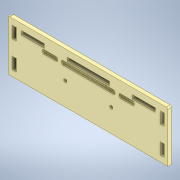
# Autodesk Inventor part: case bottom front
Saved by Autodesk Inventor 2022.3 (Build 263350030, 350C)
## iProperties
Created: 2021-05-28
Part Number: case bottom front
Material: Nylon, molybdenum disulphide
Document SubType Name: Modeling
Designer: benka
Density: 1.13 g/cm^3
Appearance: Nylon 6
Author: benka
Autodesk Inventor part; units mm, degrees
ref_plane "YZ Plane" through (0, 0, 0) normal (1, 0, 0) x (0, 1, 0)
ref_plane "XZ Plane" through (0, 0, 0) normal (0, 1, 0) x (-1, 0, 0)
ref_plane "XY Plane" through (0, 0, 0) normal (0, 0, 1) x (1, 0, 0)
sketch "Sketch1" plane through (0, 0, 0) normal (0, 0, 1) x (1, 0, 0)
  line L0 (-104.38, -32.9991) -> (103.62, -32.9991)
  line L1 (-102.38, 33.0009) -> (101.62, 33.0009)
  line L2 (57.998, 18.2189) -> (41.998, 18.2189)
  line L3 (41.998, 13.2189) -> (57.998, 13.2189)
  line L4 (-58.002, 18.2189) -> (-42.002, 18.2189)
  line L5 (-42.002, 13.2189) -> (-58.002, 13.2189)
  line L6 (32.998, 18.2189) -> (-33.002, 18.2189)
  line L7 (-33.002, 13.2189) -> (32.998, 13.2189)
  arc A0 (34.998, 16.2189) -> (32.998, 18.2189) centre (32.998, 16.2189) ccw
  arc A1 (-35.002, 15.2189) -> (-33.002, 13.2189) centre (-33.002, 15.2189) ccw
  arc A2 (-33.002, 18.2189) -> (-35.002, 16.2189) centre (-33.002, 16.2189) ccw
  arc A3 (-40.002, 16.2189) -> (-42.002, 18.2189) centre (-42.002, 16.2189) ccw
  arc A4 (-42.002, 13.2189) -> (-40.002, 15.2189) centre (-42.002, 15.2189) ccw
  arc A5 (-60.002, 15.2189) -> (-58.002, 13.2189) centre (-58.002, 15.2189) ccw
  arc A6 (-58.002, 18.2189) -> (-60.002, 16.2189) centre (-58.002, 16.2189) ccw
  arc A7 (39.998, 15.2189) -> (41.998, 13.2189) centre (41.998, 15.2189) ccw
  arc A8 (41.998, 18.2189) -> (39.998, 16.2189) centre (41.998, 16.2189) ccw
  arc A9 (59.998, 16.2189) -> (57.998, 18.2189) centre (57.998, 16.2189) ccw
  arc A10 (57.998, 13.2189) -> (59.998, 15.2189) centre (57.998, 15.2189) ccw
  arc A11 (32.998, 13.2189) -> (34.998, 15.2189) centre (32.998, 15.2189) ccw
  line L8 (59.998, 16.2189) -> (39.998, 16.2189)
  line L9 (39.998, 15.2189) -> (59.998, 15.2189)
  line L10 (34.998, 16.2189) -> (-35.002, 16.2189)
  line L11 (-35.002, 15.2189) -> (34.998, 15.2189)
  line L12 (-40.002, 16.2189) -> (-60.002, 16.2189)
  line L13 (-60.002, 15.2189) -> (-40.002, 15.2189)
  circle A12 centre (-30.002, -2.9991) radius 2
  circle A13 centre (29.998, -2.9991) radius 2
  line L14 (-104.38, 31.0009) -> (-104.38, -32.9991)
  line L15 (103.62, 31.0009) -> (103.62, -32.9991)
  arc A14 (-102.38, 33.0009) -> (-104.38, 31.0009) centre (-102.38, 31.0009) ccw
  arc A15 (103.62, 31.0009) -> (101.62, 33.0009) centre (101.62, 31.0009) ccw
  line L16 (93.998, -24.9998) -> (93.998, -10.0006)
  line L17 (93.998, -10.0006) -> (98.998, -10.0006)
  line L18 (98.998, -24.9998) -> (98.998, -10.0006)
  line L19 (93.998, -24.9998) -> (98.998, -24.9998)
  line L20 (93.998, 9.9994) -> (93.998, 25.0009)
  line L21 (93.998, 25.0009) -> (98.998, 25.0009)
  line L22 (98.998, 9.9994) -> (98.998, 25.0009)
  line L23 (93.998, 9.9994) -> (98.998, 9.9994)
  line L24 (87.498, 20.0009) -> (57.498, 20.0009)
  line L25 (57.498, 20.0009) -> (57.498, 25.0009)
  line L26 (87.498, 25.0009) -> (57.498, 25.0009)
  line L27 (87.498, 20.0009) -> (87.498, 25.0009)
  line L28 (27.498, 20.0009) -> (-27.502, 20.0009)
  line L29 (-27.502, 20.0009) -> (-27.502, 25.0009)
  line L30 (27.498, 25.0009) -> (-27.502, 25.0009)
  line L31 (27.498, 20.0009) -> (27.498, 25.0009)
  line L32 (-57.502, 20.0009) -> (-87.502, 20.0009)
  line L33 (-87.502, 20.0009) -> (-87.502, 25.0009)
  line L34 (-57.502, 25.0009) -> (-87.502, 25.0009)
  line L35 (-57.502, 20.0009) -> (-57.502, 25.0009)
  line L36 (-99.002, 9.9994) -> (-99.002, 25.0009)
  line L37 (-99.002, 25.0009) -> (-94.002, 25.0009)
  line L38 (-94.002, 9.9994) -> (-94.002, 25.0009)
  line L39 (-99.002, 9.9994) -> (-94.002, 9.9994)
  line L40 (-99.002, -24.9998) -> (-99.002, -10.0006)
  line L41 (-99.002, -10.0006) -> (-94.002, -10.0006)
  line L42 (-94.002, -24.9998) -> (-94.002, -10.0006)
  line L43 (-99.002, -24.9998) -> (-94.002, -24.9998)
  point P0 (59.998, 18.2189)
  point P1 (59.998, 13.2189)
  point P2 (-40.002, 15.2189)
  point P3 (-60.002, 16.2189)
  point P4 (59.998, 15.2189)
  point P5 (34.998, 15.2189)
  point P6 (-35.002, 16.2189)
  point P7 (-0.002, -3)
extrude "Extrusion1" add sketch "Sketch1" along normal blind 5
body "Solid1"
